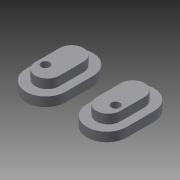
# Autodesk Inventor part: Enganche fuente
Saved by Autodesk Inventor 2014 (Build 180170000, 170)
## iProperties
Created: 2014-09-10
Part Number: Enganche fuente
Material: Generic
Document SubType Name: Modeling
Designer: Rubén
Density: 1 g/cm^3
Appearance: Default
Author: Rubén
Autodesk Inventor part; units mm, degrees
ref_plane "YZ Plane" through (0, 0, 0) normal (1, 0, 0) x (0, 1, 0)
ref_plane "XZ Plane" through (0, 0, 0) normal (0, 1, 0) x (-1, 0, 0)
ref_plane "XY Plane" through (0, 0, 0) normal (0, 0, 1) x (1, 0, 0)
sketch "Sketch1" plane through (0, 0, 0) normal (0, 1, 0) x (-1, 0, 0)
  line L0 (0, -7.9) -> (0, 7.9) construction
  line L1 (3.9, -4) -> (3.9, 4)
  line L2 (-3.9, 4) -> (-3.9, -4)
  arc A0 (-3.9, -4) -> (3.9, -4) centre (0, -4) ccw
  arc A1 (3.9, 4) -> (-3.9, 4) centre (0, 4) ccw
  line L3 (0, -11) -> (0, 11) construction
  line L4 (20, -7.9) -> (20, 7.9) construction
  line L5 (23.9, -4) -> (23.9, 4)
  line L6 (16.1, 4) -> (16.1, -4)
  arc A2 (16.1, -4) -> (23.9, -4) centre (20, -4) ccw
  arc A3 (23.9, 4) -> (16.1, 4) centre (20, 4) ccw
  line L7 (20, -11) -> (20, 11) construction
  point P0 (0, 0)
  point P1 (0, 0)
  point P2 (0, 0)
  point P3 (20, 0)
  point P4 (20, 0)
  dimension "d0" = 15.8
  dimension "d1" = 7.8
  dimension "d2" = 3.9
  dimension "d29" = 15.8
  dimension "d30" = 7.8
  dimension "d32" = 20
  dimension "d43" = 4
  dimension "d44" = 20
  dimension "d45" = 22.8254
  dimension "d46" = 20
  dimension "d47" = 11
  dimension "d48" = 0
  constraints: 24 end point, 12 point on circle, 8 point on line, 8 tangent, 4 centre point, 4 midpoint, 2 parallel, 2 vertical
  measures "d0" distance of L0.start L0.end
  measures "d1" diameter of A1
  measures "d2" distance from line of point (0, 0) L1
  measures "d29" distance of L4.start L4.end
  measures "d30" diameter of A3
  measures "d32" distance of point (20, 0) point (0, 0)
  measures "d43" distance of point (0, 0) A0.centre
  measures "d44" distance between parallel lines of L4 L0
  measures "d45" distance of L7.end point (0, 0)
  measures "d46" distance of point (20, 0) point (0, 0)
  measures "d47" distance of L3.end point (0, 0)
  measures "d48" distance of point (0, 0) point (0, 0)
extrude "Extrusion1" add sketch "Sketch1" along normal blind 6
sketch "Sketch2" plane through (0, 0, 0) normal (0, -1, 0) x (1, 0, 0)
  line L0 (0, -11) -> (0, 11) construction
  line L1 (6.5, -4.5) -> (6.5, 4.5)
  line L2 (-6.5, 4.5) -> (-6.5, -4.5)
  arc A0 (-6.5, -4.5) -> (6.5, -4.5) centre (0, -4.5) ccw
  arc A1 (6.5, 4.5) -> (-6.5, 4.5) centre (0, 4.5) ccw
  line L3 (-20, -11) -> (-20, 11) construction
  line L4 (-13.5, -4.5) -> (-13.5, 4.5)
  line L5 (-26.5, 4.5) -> (-26.5, -4.5)
  arc A2 (-26.5, -4.5) -> (-13.5, -4.5) centre (-20, -4.5) ccw
  arc A3 (-13.5, 4.5) -> (-26.5, 4.5) centre (-20, 4.5) ccw
  point P0 (0, 0)
  point P1 (0, 0)
  point P2 (-20, 0)
  dimension "d9" = 22
  dimension "d10" = 13
  dimension "d33" = 22
  dimension "d34" = 13
  dimension "d35" = 20
  constraints: 16 end point, 12 point on circle, 8 tangent, 4 centre point, 4 point on line, 2 midpoint, 2 parallel
  measures "d9" distance of L0.start L0.end
  measures "d10" diameter of A1
  measures "d33" distance of L3.start L3.end
  measures "d34" diameter of A3
  measures "d35" distance of point (0, 0) point (-20, 0)
extrude "Extrusion2" add sketch "Sketch2" against normal blind 3
sketch "Sketch3" plane through (0, 0, 0) normal (0, -1, 0) x (1, 0, 0)
  circle A0 centre (1.5, 3.1) radius 1.475
  circle A1 centre (-21.5, 3.1) radius 1.475
  point P0 (0, 0)
  point P1 (0, 3.1)
  dimension "d21" = 2.95
  dimension "d38" = 2.95
  dimension "d39" = 23
  dimension "d40" = 1.5
  dimension "d41" = 3.1
  dimension "d42" = 3.1
  constraints: 2 centre point
  measures "d21" diameter of A0
  measures "d38" diameter of A1
  measures "d39" distance of A0.centre A1.centre
  measures "d40" horizontal distance of A0.centre point (0, 0)
  measures "d41" vertical distance of A0.centre point (0, 0)
  measures "d42" vertical distance of point (0, 0) A1.centre
hole "Hole2" at (1.5, 0, 3.1) at (-21.5, 0, 3.1) direction (0, 1, 0) diameter 2.8 depth 8 tip angle 118 countersink diameter 6 countersink angle 75.6
body "Solid1"
